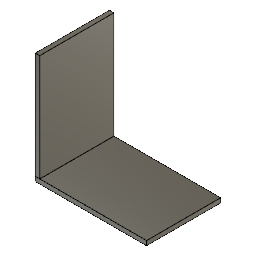
parametricBoxJoints v4 (Autodesk Fusion 360 design; units mm, degrees)
Autodesk Fusion 360 part; units mm, degrees
sketch "Sketch1" plane through (0, 0, 0) normal (0, 0, 1) x (1, 0, 0) in component "tenon"
  line L0 (0, 0) -> (304.8, 0)
  line L1 (304.8, 0) -> (304.8, 203.2)
  line L2 (304.8, 203.2) -> (0, 203.2)
  line L3 (0, 203.2) -> (0, 0)
  dimension "d1" = 304.8
  dimension "d2" = 203.2
  constraint horizontal L0
  constraint vertical L1
  constraint horizontal L2
  constraint vertical L3
  constraint coincident L0.start L3.end
  measures "d1" distance of L1.end L2.end
  measures "d2" distance of L0.end L1.end
extrude "Extrude1" add sketch "Sketch1" along normal blind 12.7 makes body 1 in component "tenon"
sketch "Sketch2" plane through (0, 0, 12.7) normal (0, 0, 1) x (-1, 0, 0) in component "tenon"
  line L0 (0, -203.2) -> (0, 0)
  line L1 (0, 0) -> (-304.8, 0)
  line L2 (-304.8, 0) -> (-304.8, -203.2)
  line L3 (-304.8, -203.2) -> (0, -203.2)
  line L4 (0, -23.9059) -> (-12.7, -23.9059)
  line L5 (-12.7, -23.9059) -> (-12.7, -11.9529)
  line L6 (-12.7, -11.9529) -> (0, -11.9529)
  line L7 (0, -11.9529) -> (0, -23.9059)
  dimension "d9" = 11.9529
  dimension "d10" = 11.9529
  dimension "d11" = 12.7
  constraint horizontal L4
  constraint vertical L5
  constraint horizontal L6
  constraint vertical L7
  constraint coincident L0 L4.start
  measures "d9" distance of L1 L6
  measures "d10" distance of L4.end L5.end
  measures "d11" distance of L4.start L4.end
extrude "Extrude2" cut sketch "Sketch2" against normal through all contours L0 L4 L5 L6 L7 bodies 1 in component "tenon"
pattern_linear "R-Pattern1" count 8 spacing 23.9059 along (0, 1, 0) of "Extrude2" in component "tenon"
sketch "Sketch1 (2)" plane through (0, 0, 0) normal (0, 0, 1) x (1, 0, 0) in component "mortise"
  line L0 (0, 0) -> (-304.8, 0)
  line L1 (-304.8, 0) -> (-304.8, 203.2)
  line L2 (-304.8, 203.2) -> (0, 203.2)
  line L3 (0, 203.2) -> (0, 0)
  dimension "d17" = 304.8
  dimension "d18" = 203.2
  constraint horizontal L0
  constraint vertical L1
  constraint horizontal L2
  constraint vertical L3
  constraint coincident L0.start L3.end
  measures "d17" distance of L0.start L0.end
  measures "d18" distance of L0.start L2.end
extrude "Extrude1'" add sketch "Sketch1 (2)" along normal blind 12.7 separate body makes body 2 in component "mortise"
sketch "Sketch2 (2)" plane through (0, 0, 12.7) normal (0, 0, 1) x (-1, 0, 0) in component "mortise"
  line L0 (0, -203.2) -> (304.8, -203.2)
  line L1 (304.8, -203.2) -> (304.8, 0)
  line L2 (304.8, 0) -> (0, 0)
  line L3 (0, 0) -> (0, -203.2)
  line L4 (0, 0) -> (12.7, 0)
  line L5 (12.7, 0) -> (12.7, -11.9529)
  line L6 (12.7, -11.9529) -> (0, -11.9529)
  line L7 (0, -11.9529) -> (0, 0)
  dimension "d21" = 12.7
  dimension "d22" = 11.9529
  constraint horizontal L4
  constraint vertical L5
  constraint horizontal L6
  constraint vertical L7
  constraint coincident L3 L2.end
  constraint coincident L2.end L3.start
  measures "d21" distance of L5.end L6.end
  measures "d22" distance of L4.end L5.end
extrude "Extrude2'" cut sketch "Sketch2 (2)" against normal through all contours L2 L3 L4 L5 L6 L7 bodies 2 in component "mortise"
pattern_linear "R-Pattern1'" count 9 spacing 23.9059 along (0, 1, 0) of "Extrude2'" in component "mortise"
component "tenon" placed x (1, 0, 0) y (0, 1, 0) z (0, 0, 1) at (0, 0, 0)
component "mortise" placed x (0, 0, -1) y (0, 1, 0) z (1, 0, 0) at (0, 0, 0)
equation "d1 = length"
equation "d2 = width"
equation "width = 8 in"
equation "length = 12 in"
equation "thick = 0.5 in"
equation "fingerNum = 8"
equation "d7 = thick"
equation "d9 = width / ( 2 * fingerNum + 1 )"
equation "d10 = width / ( 2 * fingerNum + 1 )"
equation "d11 = thick"
equation "d13 = fingerNum"
equation "d15 = -width / ( fingerNum + 0.5 )"
equation "d17 = length"
equation "d18 = width"
equation "d19 = thick"
equation "d21 = thick"
equation "d22 = width / ( 2 * fingerNum + 1 )"
equation "d24 = fingerNum + 1"
equation "d26 = width / ( fingerNum + 0.5 )"
